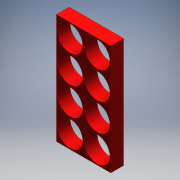
# Autodesk Inventor part: Cell_Spacer
Saved by Autodesk Inventor 2016 (Build 200138000, 138)
## iProperties
Created: 2016-04-13
Part Number: Cell_Spacer
Material: ABS Plastic
Document SubType Name: Modeling
Designer: agmle
Density: 1.06 g/cm^3
Appearance: Red
Author: agmle
Autodesk Inventor part; units mm, degrees
ref_plane "YZ Plane" through (0, 0, 0) normal (1, 0, 0) x (0, 1, 0)
ref_plane "XZ Plane" through (0, 0, 0) normal (0, 1, 0) x (-1, 0, 0)
ref_plane "XY Plane" through (0, 0, 0) normal (0, 0, 1) x (1, 0, 0)
sketch "Sketch1" plane through (0, 0, 0) normal (0, 1, 0) x (-1, 0, 0)
  line L0 (42.5, 86) -> (-42.5, 86)
  line L1 (-42.5, 86) -> (-42.5, -86)
  line L2 (-42.5, -86) -> (42.5, -86)
  line L3 (42.5, -86) -> (42.5, 86)
  line L4 (42.5, 0) -> (-42.5, 0) construction
  circle A0 centre (21.25, 64.5) radius 20
  line L5 (-21.25, 86) -> (-21.25, -86) construction
  line L6 (21.25, -86) -> (21.25, 86) construction
  circle A1 centre (21.25, 21.5) radius 20
  circle A2 centre (21.25, -21.5) radius 20
  circle A3 centre (21.25, -64.5) radius 20
  circle A4 centre (-21.25, -64.5) radius 20
  circle A5 centre (-21.25, -21.5) radius 20
  circle A6 centre (-21.25, 21.5) radius 20
  circle A7 centre (-21.25, 64.5) radius 20
  line L7 (42.5, 64.5) -> (-42.5, 64.5) construction
  line L8 (42.5, 21.5) -> (-42.5, 21.5) construction
  line L9 (42.5, -21.5) -> (-42.5, -21.5) construction
  line L10 (42.5, -64.5) -> (-42.5, -64.5) construction
  point P0 (0, 0)
  point P1 (0, 0)
  dimension "d0" = 172
  dimension "d1" = 85
  dimension "d2" = 40
  dimension "d3" = 42.5
  dimension "d4" = 21.25
  dimension "d5" = 43
  dimension "d6" = 43
  dimension "d7" = 43
  dimension "d8" = 21.5
  constraints: 28 point on line, 22 end point, 8 centre point, 7 equal radius, 7 perpendicular, 3 midpoint, 2 parallel, 1 coincident, 1 horizontal
  measures "d0" distance of L2.end L0.start
  measures "d1" distance of L0.start L0.end
  measures "d2" diameter of A0
  measures "d3" distance between parallel lines of L5 L6
  measures "d4" distance between parallel lines of L3 L6
  measures "d5" distance between parallel lines of L8 L7
  measures "d6" distance between parallel lines of L9 L8
  measures "d7" distance between parallel lines of L10 L9
  measures "d8" distance between parallel lines of L2 L10
extrude "Extrusion1" add sketch "Sketch1" along normal blind 20
equation "\"d3\" = 0.5 * d1"
equation "\"d4\" = 0.25 * d1"
equation "\"d5\" = 0.25 * d0"
equation "\"d6\" = d5"
equation "\"d7\" = d5"
equation "\"d8\" = 0.125 * d0"
body "Solid1"
